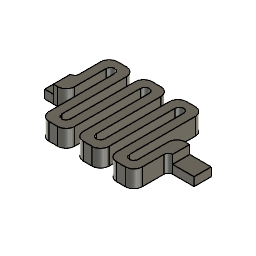
Canal - ressort v4 (Autodesk Fusion 360 design; units mm, degrees)
Autodesk Fusion 360 part; units mm, degrees
sketch "Sketch1" plane through (0, 0, 0) normal (0, 0, 1) x (1, 0, 0)
  line L0 (2.5, 5.6365) -> (1.5, 5.6365)
  line L1 (1.5, 5.6365) -> (1.5, 3.6365)
  line L2 (1.5, 3.6365) -> (2.7001, 3.6365)
  line L3 (2.7001, 3.6365) -> (3, 3.6365)
  line L4 (4, 4.6365) -> (4, 8.2817)
  line L5 (5, 8.2817) -> (5, 0.6365)
  line L6 (3, 6.1365) -> (3, 8.6365)
  line L7 (4, 9.6365) -> (5, 9.6365)
  line L8 (6, 8.6365) -> (6, 1.5003)
  arc A0 (3, 3.6365) -> (4, 4.6365) centre (3, 4.6365) ccw
  arc A1 (4, 9.6365) -> (3, 8.6365) centre (4, 8.6365) ccw
  arc A2 (6, 8.6365) -> (5, 9.6365) centre (5, 8.6365) ccw
  arc A3 (4.1477, 8.6365) -> (4, 8.2817) centre (4.5, 8.2817) ccw
  arc A4 (5, 8.2817) -> (4.1477, 8.6365) centre (4.5, 8.2817) ccw
  line L9 (6, 1.5003) -> (6, 1.1365)
  line L10 (6, -0.3635) -> (7, -0.3635)
  arc A5 (5, 0.6365) -> (6, -0.3635) centre (6, 0.6365) ccw
  arc A6 (6, 1.1365) -> (6.4999, 0.6365) centre (6.5, 1.1365) ccw
  line L11 (7, 1.1365) -> (7, 8.6365)
  arc A7 (6.4999, 0.6365) -> (7, 1.1365) centre (6.5, 1.1365) ccw
  line L12 (8, 0.6365) -> (8, 8.2817)
  arc A8 (7, -0.3635) -> (8, 0.6365) centre (7, 0.6365) ccw
  arc A9 (2.5, 5.6365) -> (3, 6.1365) centre (2.5, 6.1365) ccw
  line L13 (2.5, 5.6365) -> (2.5, 3.6365)
  arc A10 (8, 9.6365) -> (7, 8.6365) centre (8, 8.6365) ccw
  arc A11 (8.1477, 8.6365) -> (8, 8.2817) centre (8.5, 8.2817) ccw
  arc A12 (9, 8.2817) -> (8.1477, 8.6365) centre (8.5, 8.2817) ccw
  line L14 (8, 9.6365) -> (9, 9.6365)
  arc A13 (10, 8.6365) -> (9, 9.6365) centre (9, 8.6365) ccw
  line L15 (9, 8.2817) -> (9, 0.6365)
  line L16 (10, 8.6365) -> (10, 1.5003)
  line L17 (11, 1.1365) -> (11, 8.6365)
  line L18 (12, 0.6365) -> (12, 8.2817)
  arc A14 (11, -0.3635) -> (12, 0.6365) centre (11, 0.6365) ccw
  arc A15 (10.4999, 0.6365) -> (11, 1.1365) centre (10.5, 1.1365) ccw
  arc A16 (10, 1.1365) -> (10.4999, 0.6365) centre (10.5, 1.1365) ccw
  line L19 (10, 1.5003) -> (10, 1.1365)
  arc A17 (9, 0.6365) -> (10, -0.3635) centre (10, 0.6365) ccw
  line L20 (10, -0.3635) -> (11, -0.3635)
  arc A18 (12, 9.6365) -> (11, 8.6365) centre (12, 8.6365) ccw
  arc A19 (12.1477, 8.6365) -> (12, 8.2817) centre (12.5, 8.2817) ccw
  arc A20 (13, 8.2817) -> (12.1477, 8.6365) centre (12.5, 8.2817) ccw
  line L21 (12, 9.6365) -> (13, 9.6365)
  arc A21 (14, 8.6365) -> (13, 9.6365) centre (13, 8.6365) ccw
  line L22 (13, 8.2817) -> (13, 0.4991)
  line L23 (14, 8.6365) -> (14, 1.5003)
  arc A22 (15, -0.5009) -> (16, 0.4991) centre (15, 0.4991) ccw
  arc A23 (14.4999, 0.4991) -> (15, 0.9991) centre (14.5, 0.9991) ccw
  arc A24 (14, 0.9991) -> (14.4999, 0.4991) centre (14.5, 0.9991) ccw
  line L24 (14, 1.5003) -> (14, 0.9991)
  arc A25 (13, 0.4991) -> (14, -0.5009) centre (14, 0.4991) ccw
  line L25 (14, -0.5009) -> (15, -0.5009)
  line L26 (16, 0.4991) -> (16, 2.9991)
  line L27 (16.5, 3.4991) -> (19, 3.4991)
  line L28 (19, 3.4991) -> (19, 5.4991)
  line L29 (19, 5.4991) -> (16, 5.4991)
  line L30 (16.5, 3.4991) -> (16.5, 5.4991)
  line L31 (15, 4.4991) -> (15, 0.9991)
  arc A26 (16.5, 3.4991) -> (16, 2.9991) centre (16.5, 2.9991) ccw
  arc A27 (16, 5.4991) -> (15, 4.4991) centre (16, 4.4991) ccw
  point P0 (3, 5.6365)
  point P1 (5, -0.3635)
  point P2 (16, 3.4991)
  dimension "d1" = 1
  dimension "d2" = 1
  dimension "d3" = 1
  dimension "d4" = 1
  dimension "d5" = 1
  dimension "d6" = 0.5
  dimension "d8" = 4
  dimension "d9" = 1
  dimension "d10" = 0.5
  dimension "d11" = 1
  dimension "d12" = 0.5
  dimension "d13" = 1
  dimension "d14" = 1
  dimension "d15" = 1
  dimension "d17" = 1
  dimension "d18" = 2
  dimension "d37" = 0.5
  dimension "d41" = 1
  dimension "d55" = 1
  dimension "d58" = 4
  dimension "d59" = 0
  dimension "d60" = 3
  dimension "d61" = 4
  dimension "d63" = 2
  dimension "d65" = 0.5
  dimension "d66" = 1
  dimension "d69" = 3
  dimension "d70" = 2.5
  dimension "d69" = 3
  constraint horizontal L0
  constraint vertical L1
  constraint horizontal L2
  constraint perpendicular L3 L4
  constraint perpendicular L6 L7
  constraint perpendicular L7 L8
  constraint tangent L3 A0
  constraint tangent L4 A0
  constraint tangent L6 A1
  constraint tangent L7 A1
  constraint tangent L7 A2
  constraint tangent L8 A2
  constraint tangent L4 A3
  constraint tangent L5 A4
  constraint equal A3 A4
  constraint coincident A3.start A4.end
  constraint parallel L8 L9
  constraint vertical L5
  constraint perpendicular L5 L10
  constraint coincident P1 L5
  constraint coincident P1 L10
  constraint tangent L5 A5
  constraint tangent L10 A5
  constraint tangent L9 A6
  constraint tangent L11 A7
  constraint coincident A6.end A7.start
  constraint perpendicular L10 L12
  constraint tangent L10 A8
  constraint tangent L12 A8
  constraint coincident P0 L6
  constraint tangent L6 A9
  constraint coincident L0.start A9.start
  constraint coincident L2 L13.end
  constraint perpendicular L2 L13
  constraint coincident L11.end A10.end
  constraint coincident L12.end A11.end
  constraint vertical L26
  constraint perpendicular L26 L27
  constraint perpendicular L27 L28
  constraint coincident L27 L30.start
  constraint coincident L29 L30.end
  constraint perpendicular L29 L30
  constraint tangent A23 L31
  constraint coincident P2 L26
  constraint coincident P2 L27
  constraint tangent L26 A26
  constraint tangent L27 A26
  constraint tangent L29 A27
  constraint tangent L31 A27
  measures "d1" distance of L4 L6
  measures "d2" distance of L5 L8
  measures "d3" radius of A0
  measures "d4" radius of A1
  measures "d5" radius of A2
  measures "d6" radius of A3
  measures "d8" vertical distance of L2.end P1
  measures "d9" radius of A5
  measures "d10" radius of A6
  measures "d11" distance of L8 L11
  measures "d12" radius of A7
  measures "d13" distance of L11 L12
  measures "d14" radius of A8
  measures "d15" distance of L10 A6.end
  measures "d17" distance of L7 A3.start
  measures "d18" distance of L0.end L1.end
  measures "d37" radius of A9
  measures "d41" distance of L1 L13
  measures "d55" distance of L4 L5
  measures "d60" distance of A22.end P2
  measures "d61" distance of L0 L7
  measures "d63" distance of L27.end L28.end
  measures "d65" radius of A26
  measures "d66" radius of A27
  measures "d69" distance of L26 L28
  measures "d70" distance of L28 L30
extrude "Extrude6" add sketch "Sketch1" along normal blind 1 contours L0 L1 L2 L13 | L27 L28 L29 L30 makes body 1 at (2.1666, 4.3032, 0) makes body 2 at (18.1667, 4.1658, 0)
extrude "Extrude5" add sketch "Sketch1" along normal blind 2 separate body contours L2 L3 L4 L5 L6 L7 L8 A0 A1 A2 A3 A4 L9 L10 A5 A6 L11 A7 L12 A8 A9 L13 A10 A11 A12 L14 A13 L15 L16 L17 L18 A14 A15 A16 L19 A17 L20 A18 A19 A20 L21 A21 L22 L23 A22 A23 A24 L24 A25 L25 L26 L29 L30 L31 A26 A27 makes body 3
equation "d69 = 557fdcba-3344-46c9-b6e3-04745b4f979f"
